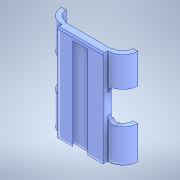
# Autodesk Inventor part: valve holder
Saved by Autodesk Inventor 2020 (Build 240168000, 168)
## iProperties
Created: 2020-02-09
Part Number: valve holder
Material: Generic
Document SubType Name: Modeling
Designer: Ball
Density: 1 g/cm^3
Appearance: Default
Author: Ball
Autodesk Inventor part; units mm, degrees
ref_plane "YZ Plane" through (0, 0, 0) normal (1, 0, 0) x (0, 1, 0)
ref_plane "XZ Plane" through (0, 0, 0) normal (0, 1, 0) x (-1, 0, 0)
ref_plane "XY Plane" through (0, 0, 0) normal (0, 0, 1) x (1, 0, 0)
sketch "Sketch1" plane through (0, 0, 0) normal (0, 1, 0) x (-1, 0, 0)
  line L0 (24.3078, -4.8641) -> (0, -4.8641)
  line L1 (24.3078, -4.8641) -> (0, 0) construction
  line L2 (0, 0) -> (24.3078, -1.2319) construction
  line L3 (0, 3.5941) -> (23.5585, 3.5941)
  line L4 (23.5585, 3.5941) -> (23.5585, -1.2319)
  line L5 (24.3078, -6.0325) -> (24.3078, -4.8515)
  arc A0 (34.7218, -16.4465) -> (24.3078, -6.0325) centre (24.3078, -16.4465) ccw
  line L6 (34.7218, -16.4465) -> (39.5224, -16.4465)
  line L7 (0, -4.8641) -> (0, 22.9231) construction
  line L8 (23.5585, -1.2319) -> (24.3078, -1.2319)
  line L9 (-24.3078, -4.8641) -> (0, -4.8641)
  line L10 (-24.3078, -4.8641) -> (0, 0) construction
  line L11 (0, 0) -> (-24.3078, 4.8641) construction
  line L12 (0, 3.5941) -> (-23.5585, 3.5941)
  line L13 (-24.3078, -6.0325) -> (-24.3078, -4.8515)
  arc A1 (-24.3078, -6.0325) -> (-34.7218, -16.4465) centre (-24.3078, -16.4465) ccw
  line L14 (-34.7218, -16.4465) -> (-39.5224, -16.4465)
  line L15 (-23.5585, 3.5941) -> (-23.5585, -1.2319)
  line L16 (-23.5585, 3.5941) -> (-18.7325, 3.5941) construction
  line L17 (-23.5585, -1.2319) -> (-24.3078, -1.2319)
  arc A2 (39.5224, -16.4465) -> (24.3078, -1.2319) centre (24.3078, -16.4465) ccw
  arc A3 (-24.3078, -1.2319) -> (-39.5224, -16.4465) centre (-24.3078, -16.4465) ccw
  point P0 (0, 0)
  dimension "d13" = 20.828
  dimension "d14" = 10.414
  dimension "d16" = 10.414
  dimension "d22" = 4.826
  dimension "d23" = 3.6322
  dimension "d25" = 4.826
  dimension "d26" = 90
  constraints: 36 end point, 8 point on circle, 4 centre point, 4 point on line, 3 horizontal, 2 coincident, 2 vertical, 1 parallel, 1 perpendicular
  measures "d13" diameter of A0
  measures "d14" distance of L5.start A0.centre
  measures "d16" distance from line of L5.start L6
  measures "d22" distance of L3.end L4.end
  measures "d23" distance between parallel lines of L0 L8
  measures "d25" distance of L12.end L15.end
  measures "d26" angle of L15 L16
extrude "Extrusion1" add sketch "Sketch1" along normal blind 108.0008
sketch "Sketch2" plane through (0, 0, 0) normal (0, -1, 0) x (1, 0, 0)
  line L0 (-23.5585, 3.5941) -> (23.5585, 3.5941) projected
  line L1 (7.62, 3.5941) -> (-7.62, 3.5941)
  line L2 (0, 0.3429) -> (12.7, 0.3429)
  line L3 (12.7, 0.3429) -> (7.62, 3.5941)
  line L4 (0, 0.3429) -> (-12.7, 0.3429)
  line L5 (-12.7, 0.3429) -> (-7.62, 3.5941)
  point P0 (0, 0)
  dimension "d29" = 15.24
  dimension "d30" = 15.9385
  dimension "d31" = 15.9385
  dimension "d35" = 25.4
  dimension "d36" = 3.2512
  constraints: 10 end point, 3 point on line, 1 horizontal
  measures "d29" distance of L1.start L1.end
  measures "d30" distance of L0.end L1.start
  measures "d31" distance of L0.start L1.end
  measures "d35" distance of L4.end L2.end
  measures "d36" distance between parallel lines of L4 L0
extrude "Extrusion2" cut sketch "Sketch2" against normal blind 94.9706
sketch "Sketch3" plane through (-34.7218, 0, -16.4465) normal (0, 0, -1) x (-1, 0, 0)
  line L0 (7.6503, 110.5775) -> (-78.6791, 110.5775)
  line L1 (-78.6791, 110.5775) -> (-78.6791, 99.187)
  line L2 (-78.6791, 99.187) -> (7.6503, 99.187)
  line L3 (7.6503, 99.187) -> (7.6503, 110.5775)
  line L4 (-27.1018, 94.9706) -> (-42.3418, 94.9706) projected
  point P0 (-34.7218, 0)
  dimension "d39" = 4.2164
  constraints: 8 end point, 2 parallel, 1 horizontal, 1 perpendicular
  measures "d39" distance between parallel lines of L2 L4
extrude "Extrusion3" cut sketch "Sketch3" against normal through all
fillet "Fillet1" radius 1.5875 1 edges at (0, 99.187, 3.5941)
sketch "Sketch5" plane through (24.3078, 99.187, -4.8641) normal (0, 0, -1) x (-1, 0, 0)
  line L0 (0.7493, -99.187) -> (0.7493, -1.5875) projected
  line L1 (0.7493, -64.897) -> (-26.6597, -64.897)
  line L2 (0, -99.187) -> (48.6156, -99.187) projected
  line L3 (-26.6597, -64.897) -> (-26.6597, -31.115)
  line L4 (-26.6597, -31.115) -> (0.7493, -31.115)
  line L5 (-26.6597, -31.115) -> (0.7493, -31.115)
  line L6 (0.7493, -31.115) -> (0.7493, -64.897)
  line L7 (0.7493, -64.897) -> (-26.6597, -64.897)
  line L8 (-26.6597, -64.897) -> (-26.6597, -31.115)
  line L9 (41.7275, -65.786) -> (92.2079, -65.786)
  line L10 (48.6156, -92.837) -> (59.0296, -92.837) projected
  line L11 (41.7275, -31.496) -> (92.2079, -31.496)
  line L12 (47.8663, -99.187) -> (47.8663, -1.5875) projected
  line L13 (47.8663, -31.496) -> (92.2079, -31.496)
  line L14 (92.2079, -31.496) -> (92.2079, -65.786)
  line L15 (92.2079, -65.786) -> (47.8663, -65.786)
  line L16 (47.8663, -65.786) -> (47.8663, -31.496)
  line L17 (59.0296, -99.187) -> (63.8302, -99.187) projected
  point P0 (24.3078, -99.187)
  point P1 (47.8663, -65.786)
  dimension "d52" = 34.29
  dimension "d53" = 33.782
  dimension "d55" = 34.29
  dimension "d59" = 33.401
  constraints: 26 end point, 5 horizontal, 4 parallel, 4 point on line, 3 perpendicular, 1 vertical
  measures "d52" distance between parallel lines of L1 L2
  measures "d53" distance of L1.end L3.end
  measures "d55" distance between parallel lines of L9 L11
  measures "d59" distance between parallel lines of L9 L17
extrude "Extrusion5" cut sketch "Sketch5" along normal through all both and the other way through all
fillet "Fillet2" radius 6.35 4 edges at (-23.5585, 67.691, -3.048) (-23.5585, 33.401, -3.048) (23.5585, 68.072, -3.048) (23.5585, 34.29, -3.048)
ref_plane "Work Plane2" through (0, 5.0038, 0) normal (0, -1, 0) x (1, 0, 0)
sketch "Sketch6" plane through (0, 5.0038, 0) normal (0, -1, 0) x (1, 0, 0)
  arc A0 (-24.3078, -4.1433) -> (-24.3078, -28.5273) centre (-24.3078, -16.3353) ccw
  arc A1 (24.3078, -28.5273) -> (24.3078, -4.1433) centre (24.3078, -16.3353) ccw
  line L0 (24.3078, -4.1433) -> (-24.3078, -4.1433)
  line L1 (-24.3078, -28.5273) -> (24.3078, -28.5273)
  point P0 (0, 0)
  point P1 (-24.3078, -4.8641)
  point P2 (24.3078, -4.8641)
  dimension "d61" = 24.384
  constraints: 4 end point, 4 point on circle, 2 centre point, 2 tangent, 1 horizontal, 1 parallel
  measures "d61" diameter of A0
extrude "Extrusion6" cut sketch "Sketch6" against normal blind 5.08
body "Solid1"
